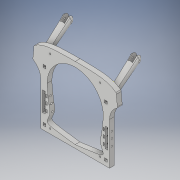
# Autodesk Inventor part: base
Saved by Autodesk Inventor 2019 (Build 230136000, 136)
## iProperties
Created: 2019-04-08
Part Number: base
Material: Ogólny
Document SubType Name: Modeling
Designer: terg
Density: 1 g/cm^3
Appearance: Domyślna
Author: terg
## iProperties of the stored document base_Drukowanie 3D.ipt
Created: 2019-04-08
Part Number: base_Drukowanie 3D
Material: Ogólny
Document SubType Name: Modeling
Designer: terg
Density: 1 g/cm^3
Appearance: Domyślna
Author: terg
Autodesk Inventor part; units mm, degrees
sketch "Szkic2" plane through (0, 0, 0) normal (0, 0, 1) x (1, 0, 0)
  line L0 (37, 65) -> (42, 65) construction
  line L1 (42, 28) -> (37, 28) construction
  line L2 (37, 65) -> (42, 65)
  line L3 (42, 65) -> (42, 28)
  line L4 (42, 28) -> (37, 28)
  line L5 (37, 28) -> (37, 65)
  line L6 (45, 80) -> (45, 0)
  line L7 (45, 0) -> (-20, 0)
  arc A0 (75, 110) -> (45, 80) centre (75, 80) ccw
  line L8 (75, 110) -> (77.9284, 114.3525) construction
  line L9 (77.9284, 114.3525) -> (81.9048, 129.5351) construction
  line L10 (81.9048, 129.5351) -> (73.952, 146.8867) construction
  line L11 (73.952, 146.8867) -> (59.3093, 153.7043) construction
  line L12 (59.3093, 153.7043) -> (47.9247, 160) construction
  line L13 (47.9247, 160) -> (-20, 160) construction
  spline S0 degree 4 poles (75, 110) (77.9284, 114.3525) (81.9048, 129.5351) (73.952, 146.8867) (59.3093, 153.7043) (47.9247, 160) (-20, 160) knots 1 1 1 1 1 2 3 4 4 4 4 4
  line L14 (0, 80) -> (0, 40) construction
  line L15 (-20, 0) -> (-20, 160) construction
  line L16 (-77, 65) -> (-82, 65) construction
  line L17 (-82, 28) -> (-77, 28) construction
  line L18 (-77, 65) -> (-82, 65)
  line L19 (-82, 65) -> (-82, 28)
  line L20 (-82, 28) -> (-77, 28)
  line L21 (-77, 28) -> (-77, 65)
  line L22 (-85, 80) -> (-85, 0)
  line L23 (-85, 0) -> (-20, 0)
  arc A1 (-85, 80) -> (-115, 110) centre (-115, 80) ccw
  line L24 (-115, 110) -> (-117.9284, 114.3525) construction
  line L25 (-117.9284, 114.3525) -> (-121.9048, 129.5351) construction
  line L26 (-121.9048, 129.5351) -> (-113.952, 146.8867) construction
  line L27 (-113.952, 146.8867) -> (-99.3093, 153.7043) construction
  line L28 (-99.3093, 153.7043) -> (-87.9247, 160) construction
  line L29 (-87.9247, 160) -> (-20, 160) construction
  spline S1 degree 4 poles (-115, 110) (-117.9284, 114.3525) (-121.9048, 129.5351) (-113.952, 146.8867) (-99.3093, 153.7043) (-87.9247, 160) (-20, 160) knots 1 1 1 1 1 2 3 4 4 4 4 4
  line L30 (-40, 80) -> (-40, 40) construction
  dimension "d23" = 30
  dimension "d24" = 65
  constraints: 38 end point, 21 symmetric about line, 8 coincident, 4 point on circle, 3 horizontal, 3 parallel, 2 centre point, 2 vertical, 1 perpendicular, 7 other
  measures "d23" radius of A0
  measures "d24" distance of L6.end L7.end
extrude "Wyciągnięcie proste1" add sketch "Szkic2" along normal blind 9
sketch "Szkic3" plane through (0, 0, 9) normal (0, 0, 1) x (1, 0, 0)
  line L0 (-85, 0) -> (45, 0) projected
  line L1 (-20, 0) -> (-67.244, 0)
  line L2 (-67.244, 0) -> (27.244, 0)
  circle A0 centre (-67.244, 8.994) radius 1.5
  circle A1 centre (27.244, 10) radius 1.5
  circle A2 centre (-67.244, 131.168) radius 1.5
  circle A3 centre (27.244, 131.168) radius 1.5
  point P0 (0, 0)
  dimension "d29" = 3
  dimension "d30" = 3
  dimension "d32" = 3
  dimension "d33" = 3
  constraints: 6 coincident, 4 centre point, 4 end point, 2 point on line, 1 midpoint
  measures "d29" diameter of A0
  measures "d30" diameter of A1
  measures "d32" diameter of A2
  measures "d33" diameter of A3
sketch "Szkic4" plane through (0, 0, 9) normal (0, 0, 1) x (1, 0, 0)
  line L0 (-85, 0) -> (45, 0) construction
  line L1 (-20, 0) -> (-20, 160) construction
  arc A0 (33.1064, 80) -> (-73.1064, 80) centre (-20, 80) ccw
  line L2 (-73.1064, 80) -> (-75.9423, 68.2413) construction
  line L3 (-75.9423, 68.2413) -> (-69.081, 45.3704) construction
  line L4 (-69.081, 45.3704) -> (-64.3162, 33.5537) construction
  line L5 (-64.3162, 33.5537) -> (-75.1799, 18.6876) construction
  line L6 (-75.1799, 18.6876) -> (-73.1064, 12.7793) construction
  line L7 (-73.1064, 12.7793) -> (-51.356, 10.6828) construction
  line L8 (-51.356, 10.6828) -> (-23.7203, 6.2992) construction
  line L9 (-23.7203, 6.2992) -> (-20, 6.2992) construction
  spline S0 degree 4 poles (-73.1064, 80) (-75.9423, 68.2413) (-69.081, 45.3704) (-64.3162, 33.5537) (-75.1799, 18.6876) (-73.1064, 12.7793) (-51.356, 10.6828) (-23.7203, 6.2992) (-20, 6.2992) knots 1 1 1 1 1 2 3 4 5 6 6 6 6 6
  line L10 (33.1064, 80) -> (35.9423, 68.2413) construction
  line L11 (35.9423, 68.2413) -> (29.081, 45.3704) construction
  line L12 (29.081, 45.3704) -> (24.3162, 33.5537) construction
  line L13 (24.3162, 33.5537) -> (35.1799, 18.6876) construction
  line L14 (35.1799, 18.6876) -> (33.1064, 12.7793) construction
  line L15 (33.1064, 12.7793) -> (11.356, 10.6828) construction
  line L16 (11.356, 10.6828) -> (-16.2797, 6.2992) construction
  line L17 (-16.2797, 6.2992) -> (-20, 6.2992) construction
  spline S1 degree 4 poles (33.1064, 80) (35.9423, 68.2413) (29.081, 45.3704) (24.3162, 33.5537) (35.1799, 18.6876) (33.1064, 12.7793) (11.356, 10.6828) (-16.2797, 6.2992) (-20, 6.2992) knots 1 1 1 1 1 2 3 4 5 6 6 6 6 6
  point P0 (0, 0)
  dimension "d34" = 160
  constraints: 7 symmetric about line, 2 end point, 2 midpoint, 2 point on circle, 1 centre point, 1 coincident, 1 perpendicular, 1 point on line, 1 vertical, 6 other
  measures "d34" distance of L1.start L1.end
extrude "Wyciągnięcie proste2" cut sketch "Szkic4" against normal blind 9
extrude "Wyciągnięcie proste3" cut sketch "Szkic3" against normal blind 9
sketch "Szkic5" plane through (0, 0, 9) normal (0, 0, 1) x (1, 0, 0)
  line L0 (-20, 160) -> (-20, 77.8902) construction
  line L1 (-20, 155) -> (-42.2049, 155) construction
  line L2 (-42.2049, 155) -> (-65.7509, 155) construction
  line L3 (-65.7509, 155) -> (-78.0422, 153.5632) construction
  line L4 (-78.0422, 153.5632) -> (-90.9908, 151.4994) construction
  line L5 (-90.9908, 151.4994) -> (-102.4767, 146.7512) construction
  line L6 (-102.4767, 146.7512) -> (-110.6216, 138.1137) construction
  line L7 (-110.6216, 138.1137) -> (-114.9161, 129.1287) construction
  line L8 (-114.9161, 129.1287) -> (-113.1391, 120.6877) construction
  line L9 (-113.1391, 120.6877) -> (-110.6216, 115.3565) construction
  spline S0 degree 4 poles (-20, 155) (-42.2049, 155) (-65.7509, 155) (-78.0422, 153.5632) (-90.9908, 151.4994) (-102.4767, 146.7512) (-110.6216, 138.1137) (-114.9161, 129.1287) (-113.1391, 120.6877) (-110.6216, 115.3565) knots 1 1 1 1 1 2 3 4 5 6 7 7 7 7 7
  line L10 (-110.6216, 115.3565) -> (-100.7117, 110.6199) construction
  line L11 (-100.7117, 110.6199) -> (-100.7117, 112.6806) construction
  line L12 (-100.7117, 112.6806) -> (-104.521, 114.5013) construction
  line L13 (-104.521, 114.5013) -> (-105.8067, 117.6302) construction
  line L14 (-105.8067, 117.6302) -> (-102.4767, 127.3399) construction
  line L15 (-102.4767, 127.3399) -> (-87.3718, 136.9774) construction
  line L16 (-87.3718, 136.9774) -> (-70.3325, 140.9019) construction
  line L17 (-70.3325, 140.9019) -> (-54.5401, 141.8394) construction
  line L18 (-54.5401, 141.8394) -> (-35.9852, 142.4325) construction
  line L19 (-35.9852, 142.4325) -> (-20, 142.4325) construction
  spline S1 degree 4 poles (-110.6216, 115.3565) (-100.7117, 110.6199) (-100.7117, 112.6806) (-104.521, 114.5013) (-105.8067, 117.6302) (-102.4767, 127.3399) (-87.3718, 136.9774) (-70.3325, 140.9019) (-54.5401, 141.8394) (-35.9852, 142.4325) (-20, 142.4325) knots 1 1 1 1 1 2 3 4 5 6 7 8 8 8 8 8
  line L20 (-20, 155) -> (2.2049, 155) construction
  line L21 (2.2049, 155) -> (25.7509, 155) construction
  line L22 (25.7509, 155) -> (38.0422, 153.5632) construction
  line L23 (38.0422, 153.5632) -> (50.9908, 151.4994) construction
  line L24 (50.9908, 151.4994) -> (62.4767, 146.7512) construction
  line L25 (62.4767, 146.7512) -> (70.6216, 138.1137) construction
  line L26 (70.6216, 138.1137) -> (74.9161, 129.1287) construction
  line L27 (74.9161, 129.1287) -> (73.1391, 120.6877) construction
  line L28 (73.1391, 120.6877) -> (70.6216, 115.3565) construction
  spline S2 degree 4 poles (-20, 155) (2.2049, 155) (25.7509, 155) (38.0422, 153.5632) (50.9908, 151.4994) (62.4767, 146.7512) (70.6216, 138.1137) (74.9161, 129.1287) (73.1391, 120.6877) (70.6216, 115.3565) knots 1 1 1 1 1 2 3 4 5 6 7 7 7 7 7
  line L29 (70.6216, 115.3565) -> (60.7117, 110.6199) construction
  line L30 (60.7117, 110.6199) -> (60.7117, 112.6806) construction
  line L31 (60.7117, 112.6806) -> (64.521, 114.5013) construction
  line L32 (64.521, 114.5013) -> (65.8067, 117.6302) construction
  line L33 (65.8067, 117.6302) -> (62.4767, 127.3399) construction
  line L34 (62.4767, 127.3399) -> (47.3718, 136.9774) construction
  line L35 (47.3718, 136.9774) -> (30.3325, 140.9019) construction
  line L36 (30.3325, 140.9019) -> (14.5401, 141.8394) construction
  line L37 (14.5401, 141.8394) -> (-4.0148, 142.4325) construction
  line L38 (-4.0148, 142.4325) -> (-20, 142.4325) construction
  spline S3 degree 4 poles (70.6216, 115.3565) (60.7117, 110.6199) (60.7117, 112.6806) (64.521, 114.5013) (65.8067, 117.6302) (62.4767, 127.3399) (47.3718, 136.9774) (30.3325, 140.9019) (14.5401, 141.8394) (-4.0148, 142.4325) (-20, 142.4325) knots 1 1 1 1 1 2 3 4 5 6 7 8 8 8 8 8
  point P0 (0, 0)
  constraints: 18 symmetric about line, 2 end point, 2 perpendicular, 2 point on line, 2 vertical, 12 other
extrude "Wyciągnięcie proste4" cut sketch "Szkic5" against normal blind 9
sketch "Szkic6" plane through (45, 0, 0) normal (1, 0, 0) x (0, 0, -1)
  line L0 (-9, 28) -> (-9, 65) projected
  line L1 (0, 65) -> (0, 28) projected
  line L2 (0, 28) -> (-9, 28) construction
  line L3 (-9, 28) -> (0, 28) construction
  line L4 (0, 65) -> (-9, 65) construction
  line L5 (0, 65) -> (-9, 65) construction
  line L6 (-4.5, 28) -> (-4.5, 34) construction
  circle A0 centre (-4.5, 34) radius 1.5
  line L7 (-4.5, 34) -> (-4.5, 46.5) construction
  circle A1 centre (-4.5, 46.5) radius 1.5
  line L8 (-4.5, 46.5) -> (-4.5, 58.5) construction
  circle A2 centre (-4.5, 58.5) radius 1.5
  point P0 (0, 0)
  dimension "d41" = 6
  dimension "d42" = 3
  dimension "d43" = 12.5
  dimension "d44" = 3
  dimension "d45" = 12
  dimension "d46" = 3
  constraints: 10 end point, 3 centre point, 3 coincident, 3 vertical, 1 collinear, 1 horizontal, 1 midpoint
  measures "d41" distance of L6.start L6.end
  measures "d42" diameter of A0
  measures "d43" distance of L7.start L7.end
  measures "d44" diameter of A1
  measures "d45" distance of L8.start L8.end
  measures "d46" diameter of A2
extrude "Wyciągnięcie proste5" cut sketch "Szkic6" against normal blind 11
ref_plane "Płaszczyzna konstrukcyjna1" through (-20, 0, 0) normal (1, 0, 0) x (0, 1, 0)
mirror "Odbij1" about plane through (-20, 0, 0) normal (1, 0, 0) of "Wyciągnięcie proste5"
sketch "Szkic7" plane through (0, 0, 9) normal (0, 0, 1) x (1, 0, 0)
  line L0 (37, 35.5) -> (37, 32.5) projected
  line L1 (37, 48) -> (37, 45) projected
  line L2 (37, 60) -> (37, 57) projected
  line L3 (37, 58.5) -> (27.7533, 58.5) construction
  line L4 (37, 46.5) -> (27.7533, 46.5) construction
  line L5 (37, 34) -> (27.7533, 34) construction
  line L6 (33.1, 43.75) -> (35.4, 43.75)
  line L7 (35.4, 43.75) -> (35.4, 49.25)
  line L8 (35.4, 49.25) -> (33.1, 49.25)
  line L9 (33.1, 49.25) -> (33.1, 43.75)
  line L10 (33.1, 43.75) -> (35.4, 49.25) construction
  line L11 (35.4, 43.75) -> (33.1, 49.25) construction
  line L12 (33.1, 31.25) -> (35.4, 31.25)
  line L13 (35.4, 31.25) -> (35.4, 36.75)
  line L14 (35.4, 36.75) -> (33.1, 36.75)
  line L15 (33.1, 36.75) -> (33.1, 31.25)
  line L16 (33.1, 31.25) -> (35.4, 36.75) construction
  line L17 (35.4, 31.25) -> (33.1, 36.75) construction
  line L18 (33, 55.75) -> (35.5, 55.75)
  line L19 (35.5, 55.75) -> (35.5, 61.25)
  line L20 (35.5, 61.25) -> (33, 61.25)
  line L21 (33, 61.25) -> (33, 55.75)
  line L22 (33, 55.75) -> (35.5, 61.25) construction
  line L23 (35.5, 55.75) -> (33, 61.25) construction
  spline S0 degree 4 poles (33.1064, 80) (35.9423, 68.2413) (29.081, 45.3704) (24.3162, 33.5537) (35.1799, 18.6876) (33.1064, 12.7793) (11.356, 10.6828) (-16.2797, 6.2992) (-20, 6.2992) knots 0 0 0 0 0 0.2 0.4 0.6 0.8 1 1 1 1 1 projected
  line L24 (29.4637, 46.5) -> (30.5401, 52.1183) construction
  line L25 (30.5401, 52.1183) -> (31.3941, 62.4324) construction
  line L26 (31.3941, 62.4324) -> (33.1064, 73.5348) construction
  line L27 (33.1064, 73.5348) -> (33.1064, 80) construction
  spline S1 degree 4 poles (29.4637, 46.5) (30.5401, 52.1183) (31.3941, 62.4324) (33.1064, 73.5348) (33.1064, 80) knots 1 1 1 1 1 2 2 2 2 2
  point P0 (0, 0)
  point P1 (34.25, 58.5)
  point P2 (34.25, 46.5)
  point P3 (34.25, 34)
  dimension "d50" = 2.3
  dimension "d51" = 5.5
  dimension "d52" = 2.3
  dimension "d53" = 5.5
  dimension "d54" = 2.5
  dimension "d55" = 5.5
  constraints: 42 end point, 9 midpoint, 6 horizontal, 6 parallel, 4 point on line, 3 perpendicular, 1 coincident, 1 vertical, 6 other
  measures "d50" distance of L8.end L7.end
  measures "d51" distance of L7.end L6.end
  measures "d52" distance of L14.end L13.end
  measures "d53" distance of L13.end L12.end
  measures "d54" distance of L20.end L19.end
  measures "d55" distance of L19.end L18.end
extrude "Wyciągnięcie proste6" add sketch "Szkic7" against normal blind 9 contours S0 S1 L20 L21 | L21 L20 S0
extrude "Wyciągnięcie proste7" cut sketch "Szkic7" against normal blind 9 contours L9 L8 L7 L6 | L15 L14 L13 L12 | L21 S0 L20 L19 L18 | L21 L20 S0
sketch "Szkic8" plane through (45, 0, 0) normal (1, 0, 0) x (0, 0, -1)
  circle A0 centre (-4.5, 34) radius 1.5 projected
  circle A1 centre (-4.5, 46.5) radius 1.5 projected
  circle A2 centre (-4.5, 58.5) radius 1.5 projected
  point P0 (0, 0)
extrude "Wyciągnięcie proste8" cut sketch "Szkic8" against normal blind 20
mirror "Odbij2" about plane through (-20, 0, 0) normal (1, 0, 0) of "Wyciągnięcie proste6", "Wyciągnięcie proste7", "Wyciągnięcie proste8"
sketch "Szkic9" plane through (0, 0, 0) normal (0, 0, -1) x (-1, 0, 0)
  line L0 (75.4, 36.75) -> (75.4, 31.25) construction
  line L1 (75.4, 31.25) -> (73.1, 31.25) construction
  line L2 (73.1, 31.25) -> (73.1, 36.75) construction
  line L3 (73.1, 36.75) -> (75.4, 36.75) construction
  line L4 (75.4, 49.25) -> (75.4, 43.75) construction
  line L5 (75.4, 43.75) -> (73.1, 43.75) construction
  line L6 (73.1, 43.75) -> (73.1, 49.25) construction
  line L7 (73.1, 49.25) -> (75.4, 49.25) construction
  line L8 (75.5, 61.25) -> (75.5, 55.75) construction
  line L9 (75.5, 55.75) -> (73, 55.75) construction
  line L10 (73, 55.75) -> (73, 61.25) construction
  line L11 (73, 61.25) -> (75.5, 61.25) construction
  line L12 (-35.5, 55.75) -> (-35.5, 61.25) construction
  line L13 (-35.5, 61.25) -> (-33, 61.25) construction
  line L14 (-33, 61.25) -> (-33, 55.75) construction
  line L15 (-33, 55.75) -> (-35.5, 55.75) construction
  line L16 (-35.4, 43.75) -> (-35.4, 49.25) construction
  line L17 (-35.4, 49.25) -> (-33.1, 49.25) construction
  line L18 (-33.1, 49.25) -> (-33.1, 43.75) construction
  line L19 (-33.1, 43.75) -> (-35.4, 43.75) construction
  line L20 (-35.4, 31.25) -> (-35.4, 36.75) construction
  line L21 (-35.4, 36.75) -> (-33.1, 36.75) construction
  line L22 (-33.1, 36.75) -> (-33.1, 31.25) construction
  line L23 (-33.1, 31.25) -> (-35.4, 31.25) construction
  circle A0 centre (67.244, 131.168) radius 1.5 construction
  circle A1 centre (67.244, 8.994) radius 1.5 construction
  circle A2 centre (-27.244, 10) radius 1.5 construction
  circle A3 centre (-27.244, 131.168) radius 1.5 construction
  arc A4 (73.1064, 80) -> (-33.1064, 80) centre (20, 80) ccw construction
  line L24 (77, 28) -> (77, 65) construction
  line L25 (77, 65) -> (82, 65) construction
  line L26 (82, 65) -> (82, 28) construction
  line L27 (82, 28) -> (77, 28) construction
  line L28 (-42, 28) -> (-42, 65) construction
  line L29 (-42, 65) -> (-37, 65) construction
  line L30 (-37, 65) -> (-37, 28) construction
  line L31 (-37, 28) -> (-42, 28) construction
  line L32 (85, 0) -> (-45, 0) construction
  line L33 (85, 80) -> (85, 0) construction
  arc A5 (115, 110) -> (85, 80) centre (115, 80) ccw construction
  arc A6 (-45, 80) -> (-75, 110) centre (-75, 80) ccw construction
  line L34 (-45, 0) -> (-45, 80) construction
  line L35 (-49.3106, 116.6116) -> (-39.3106, 116.6116)
  line L36 (-39.3106, 116.6116) -> (-39.3106, 126.6116)
  line L37 (-39.3106, 126.6116) -> (-49.3106, 126.6116)
  line L38 (-49.3106, 126.6116) -> (-49.3106, 116.6116)
  line L39 (-49.3106, 116.6116) -> (-39.3106, 126.6116) construction
  line L40 (-39.3106, 116.6116) -> (-49.3106, 126.6116) construction
  point P0 (0, 0)
  point P1 (-44.3106, 121.6116)
  dimension "d62" = 10
  dimension "d63" = 10
  constraints: 12 end point, 2 midpoint, 2 parallel, 1 horizontal, 1 perpendicular, 10 other
  measures "d62" distance of L37.end L36.end
  measures "d63" distance of L36.end L35.end
ref_plane "Płaszczyzna konstrukcyjna3" through (0, 0, -39.5) normal (0, 0, -1) x (-1, 0, 0)
ref_plane "Płaszczyzna konstrukcyjna5" through (52.8106, 146.0683, -39.5) normal (0, 0, -1) x (-1, 0, 0)
sketch "Szkic12" plane through (52.8106, 146.0683, -39.5) normal (0, 0, -1) x (-1, 0, 0)
  line L0 (0, 0) -> (17, 0) projected
  line L1 (17, 0) -> (17, 17) projected
  line L2 (17, 17) -> (0, 17) projected
  line L3 (0, 17) -> (0, 0) projected
  line L4 (0, 0) -> (17, 0) projected
  line L5 (8.5, 0) -> (8.5, 17)
  arc A0 (8.5, 0) -> (8.5, 17) centre (8.5, 8.5) ccw
  point P0 (52.8106, -146.0683)
  constraints: 2 end point, 2 midpoint, 2 point on circle, 1 centre point, 1 tangent
revolve "Obrót1" add sketch "Szkic12" angle 180 about axis through (44.3106, 146.0683, -39.5) along (0, -1, 0) contours L5 A0
loft "Wyciągnięcie złożone2" add profiles "Szkic9" section 2 edges at (35.8106, 154.5683, -39.5) (52.8106, 154.5683, -39.5)
mirror "Odbij3" about plane through (-20, 0, 0) normal (1, 0, 0) of "Wyciągnięcie złożone2", "Obrót1"
sketch "Szkic13" plane through (0, 0, 9) normal (0, 0, 1) x (1, 0, 0)
  line L0 (-89.3106, 116.6116) -> (-79.3106, 116.6116) projected
  line L1 (-79.3106, 116.6116) -> (-79.3106, 126.6116) projected
  line L2 (-79.3106, 126.6116) -> (-89.3106, 126.6116) projected
  line L3 (-89.3106, 126.6116) -> (-89.3106, 116.6116) projected
  line L4 (39.3106, 116.6116) -> (49.3106, 116.6116) projected
  line L5 (49.3106, 116.6116) -> (49.3106, 126.6116) projected
  line L6 (49.3106, 126.6116) -> (39.3106, 126.6116) projected
  line L7 (39.3106, 126.6116) -> (39.3106, 116.6116) projected
  line L8 (-75.4, 36.75) -> (-75.4, 31.25) projected
  line L9 (-75.4, 31.25) -> (-73.1, 31.25) projected
  line L10 (-73.1, 31.25) -> (-73.1, 36.75) projected
  line L11 (-73.1, 36.75) -> (-75.4, 36.75) projected
  line L12 (-75.4, 49.25) -> (-75.4, 43.75) projected
  line L13 (-75.4, 43.75) -> (-73.1, 43.75) projected
  line L14 (-73.1, 43.75) -> (-73.1, 49.25) projected
  line L15 (-73.1, 49.25) -> (-75.4, 49.25) projected
  line L16 (-75.5, 61.25) -> (-75.5, 55.75) projected
  line L17 (-75.5, 55.75) -> (-73, 55.75) projected
  line L18 (-73, 55.75) -> (-73, 61.25) projected
  line L19 (-73, 61.25) -> (-75.5, 61.25) projected
  line L20 (35.5, 55.75) -> (35.5, 61.25) projected
  line L21 (35.5, 61.25) -> (33, 61.25) projected
  line L22 (33, 61.25) -> (33, 55.75) projected
  line L23 (33, 55.75) -> (35.5, 55.75) projected
  line L24 (35.4, 43.75) -> (35.4, 49.25) projected
  line L25 (35.4, 49.25) -> (33.1, 49.25) projected
  line L26 (33.1, 49.25) -> (33.1, 43.75) projected
  line L27 (33.1, 43.75) -> (35.4, 43.75) projected
  line L28 (35.4, 31.25) -> (35.4, 36.75) projected
  line L29 (35.4, 36.75) -> (33.1, 36.75) projected
  line L30 (33.1, 36.75) -> (33.1, 31.25) projected
  line L31 (33.1, 31.25) -> (35.4, 31.25) projected
  circle A0 centre (-67.244, 131.168) radius 1.5 projected
  circle A1 centre (-67.244, 8.994) radius 1.5 projected
  circle A2 centre (27.244, 10) radius 1.5 projected
  circle A3 centre (27.244, 131.168) radius 1.5 projected
  arc A4 (33.1064, 80) -> (-73.1064, 80) centre (-20, 80) ccw projected
  line L32 (-77, 28) -> (-77, 65) projected
  line L33 (-77, 65) -> (-82, 65) projected
  line L34 (-82, 65) -> (-82, 28) projected
  line L35 (-82, 28) -> (-77, 28) projected
  line L36 (42, 28) -> (42, 65) projected
  line L37 (42, 65) -> (37, 65) projected
  line L38 (37, 65) -> (37, 28) projected
  line L39 (37, 28) -> (42, 28) projected
  line L40 (-85, 0) -> (45, 0) projected
  line L41 (-85, 80) -> (-85, 0) projected
  arc A5 (-85, 80) -> (-115, 110) centre (-115, 80) ccw projected
  arc A6 (75, 110) -> (45, 80) centre (75, 80) ccw projected
  line L42 (45, 0) -> (45, 80) projected
  line L43 (-75.4, 31.25) -> (-75.4, 36.75) projected
  line L44 (-75.4, 36.75) -> (-73.1, 36.75) projected
  line L45 (-73.1, 36.75) -> (-73.1, 31.25) projected
  line L46 (-73.1, 31.25) -> (-75.4, 31.25) projected
  line L47 (-75.4, 43.75) -> (-75.4, 49.25) projected
  line L48 (-75.4, 49.25) -> (-73.1, 49.25) projected
  line L49 (-73.1, 49.25) -> (-73.1, 43.75) projected
  line L50 (-73.1, 43.75) -> (-75.4, 43.75) projected
  line L51 (-75.5, 55.75) -> (-75.5, 61.25) projected
  line L52 (-75.5, 61.25) -> (-73, 61.25) projected
  line L53 (-73, 61.25) -> (-73, 55.75) projected
  line L54 (-73, 55.75) -> (-75.5, 55.75) projected
  line L55 (35.5, 61.25) -> (35.5, 55.75) projected
  line L56 (35.5, 55.75) -> (33, 55.75) projected
  line L57 (33, 55.75) -> (33, 61.25) projected
  line L58 (33, 61.25) -> (35.5, 61.25) projected
  line L59 (35.4, 49.25) -> (35.4, 43.75) projected
  line L60 (35.4, 43.75) -> (33.1, 43.75) projected
  line L61 (33.1, 43.75) -> (33.1, 49.25) projected
  line L62 (33.1, 49.25) -> (35.4, 49.25) projected
  line L63 (35.4, 36.75) -> (35.4, 31.25) projected
  line L64 (35.4, 31.25) -> (33.1, 31.25) projected
  line L65 (33.1, 31.25) -> (33.1, 36.75) projected
  line L66 (33.1, 36.75) -> (35.4, 36.75) projected
  circle A7 centre (-67.244, 131.168) radius 1.5 projected
  circle A8 centre (-67.244, 8.994) radius 1.5 projected
  circle A9 centre (27.244, 10) radius 1.5 projected
  circle A10 centre (27.244, 131.168) radius 1.5 projected
  arc A11 (33.1064, 80) -> (-73.1064, 80) centre (-20, 80) ccw projected
  line L67 (-77, 65) -> (-77, 28) projected
  line L68 (-77, 28) -> (-82, 28) projected
  line L69 (-82, 28) -> (-82, 65) projected
  line L70 (-82, 65) -> (-77, 65) projected
  line L71 (42, 65) -> (42, 28) projected
  line L72 (42, 28) -> (37, 28) projected
  line L73 (37, 28) -> (37, 65) projected
  line L74 (37, 65) -> (42, 65) projected
  line L75 (-85, 0) -> (45, 0) projected
  line L76 (45, 0) -> (45, 80) projected
  arc A12 (75, 110) -> (45, 80) centre (75, 80) ccw projected
  arc A13 (-85, 80) -> (-115, 110) centre (-115, 80) ccw projected
  line L77 (-85, 80) -> (-85, 0) projected
  line L78 (45, 0) -> (38, 0) construction
  line L79 (38, 0) -> (38, 10) construction
  line L80 (38, 10) -> (45, 10) construction
  line L81 (45, 10) -> (45, 0) construction
  line L82 (35.5, 12.5) -> (40.5, 12.5)
  line L83 (40.5, 12.5) -> (40.5, 7.5)
  line L84 (40.5, 7.5) -> (35.5, 7.5)
  line L85 (35.5, 7.5) -> (35.5, 12.5)
  line L86 (35.5, 12.5) -> (40.5, 7.5) construction
  line L87 (40.5, 12.5) -> (35.5, 7.5) construction
  line L88 (38, 10) -> (38, 105) construction
  line L89 (35.5, 107.5) -> (40.5, 107.5)
  line L90 (40.5, 107.5) -> (40.5, 102.5)
  line L91 (40.5, 102.5) -> (35.5, 102.5)
  line L92 (35.5, 102.5) -> (35.5, 107.5)
  line L93 (35.5, 107.5) -> (40.5, 102.5) construction
  line L94 (40.5, 107.5) -> (35.5, 102.5) construction
  point P0 (0, 0)
  dimension "d79" = 7
  dimension "d80" = 10
  dimension "d81" = 5
  dimension "d82" = 5
  dimension "d83" = 95
  dimension "d84" = 5
  dimension "d85" = 5
  constraints: 34 end point, 6 parallel, 4 midpoint, 3 horizontal, 3 perpendicular, 1 vertical, 20 other
  measures "d79" distance of L79.end L80.end
  measures "d80" distance of L78.end L79.end
  measures "d81" distance of L83.end L84.end
  measures "d82" distance of L82.end L83.end
  measures "d83" distance of L79.end L88.end
  measures "d84" distance of L90.end L91.end
  measures "d85" distance of L89.end L90.end
extrude "Wyciągnięcie proste9" cut sketch "Szkic13" against normal blind 20 contours L82 L83 L84 L85 | L89 L90 L91 L92
mirror "Odbij4" about plane through (-20, 0, 0) normal (1, 0, 0) of "Wyciągnięcie proste9"
sketch "Szkic14" plane through (0, 0, 0) normal (0, 0, -1) x (-1, 0, 0)
  point P0 (0, 0)
sketch "Szkic15" plane through (0, 0, 0) normal (0, 0, -1) x (-1, 0, 0)
  line L0 (75.5, 7.5) -> (75.5, 12.5) projected
  line L1 (75.5, 12.5) -> (80.5, 12.5) projected
  line L2 (80.5, 12.5) -> (80.5, 7.5) projected
  line L3 (80.5, 7.5) -> (75.5, 7.5) projected
  line L4 (75.5, 102.5) -> (75.5, 107.5) projected
  line L5 (75.5, 107.5) -> (80.5, 107.5) projected
  line L6 (80.5, 107.5) -> (80.5, 102.5) projected
  line L7 (80.5, 102.5) -> (75.5, 102.5) projected
  line L8 (-35.5, 12.5) -> (-35.5, 7.5) projected
  line L9 (-35.5, 7.5) -> (-40.5, 7.5) projected
  line L10 (-40.5, 7.5) -> (-40.5, 12.5) projected
  line L11 (-40.5, 12.5) -> (-35.5, 12.5) projected
  line L12 (-35.5, 107.5) -> (-35.5, 102.5) projected
  line L13 (-35.5, 102.5) -> (-40.5, 102.5) projected
  line L14 (-40.5, 102.5) -> (-40.5, 107.5) projected
  line L15 (-40.5, 107.5) -> (-35.5, 107.5) projected
  line L16 (75.4, 36.75) -> (75.4, 31.25) projected
  line L17 (75.4, 31.25) -> (73.1, 31.25) projected
  line L18 (73.1, 31.25) -> (73.1, 36.75) projected
  line L19 (73.1, 36.75) -> (75.4, 36.75) projected
  line L20 (75.4, 49.25) -> (75.4, 43.75) projected
  line L21 (75.4, 43.75) -> (73.1, 43.75) projected
  line L22 (73.1, 43.75) -> (73.1, 49.25) projected
  line L23 (73.1, 49.25) -> (75.4, 49.25) projected
  line L24 (75.5, 61.25) -> (75.5, 55.75) projected
  line L25 (75.5, 55.75) -> (73, 55.75) projected
  line L26 (73, 55.75) -> (73, 61.25) projected
  line L27 (73, 61.25) -> (75.5, 61.25) projected
  line L28 (-35.5, 55.75) -> (-35.5, 61.25) projected
  line L29 (-35.5, 61.25) -> (-33, 61.25) projected
  line L30 (-33, 61.25) -> (-33, 55.75) projected
  line L31 (-33, 55.75) -> (-35.5, 55.75) projected
  line L32 (-35.4, 43.75) -> (-35.4, 49.25) projected
  line L33 (-35.4, 49.25) -> (-33.1, 49.25) projected
  line L34 (-33.1, 49.25) -> (-33.1, 43.75) projected
  line L35 (-33.1, 43.75) -> (-35.4, 43.75) projected
  line L36 (-35.4, 31.25) -> (-35.4, 36.75) projected
  line L37 (-35.4, 36.75) -> (-33.1, 36.75) projected
  line L38 (-33.1, 36.75) -> (-33.1, 31.25) projected
  line L39 (-33.1, 31.25) -> (-35.4, 31.25) projected
  circle A0 centre (67.244, 131.168) radius 1.5 projected
  circle A1 centre (67.244, 8.994) radius 1.5 projected
  circle A2 centre (-27.244, 10) radius 1.5 projected
  circle A3 centre (-27.244, 131.168) radius 1.5 projected
  arc A4 (73.1064, 80) -> (-33.1064, 80) centre (20, 80) ccw projected
  line L40 (77, 28) -> (77, 65) projected
  line L41 (77, 65) -> (82, 65) projected
  line L42 (82, 65) -> (82, 28) projected
  line L43 (82, 28) -> (77, 28) projected
  line L44 (-42, 28) -> (-42, 65) projected
  line L45 (-42, 65) -> (-37, 65) projected
  line L46 (-37, 65) -> (-37, 28) projected
  line L47 (-37, 28) -> (-42, 28) projected
  line L48 (85, 0) -> (-45, 0) projected
  line L49 (85, 80) -> (85, 0) projected
  arc A5 (115, 110) -> (85, 80) centre (115, 80) ccw projected
  spline S0 degree 4 poles (-75, 110) (-77.9284, 114.3525) (-81.9048, 129.5351) (-73.952, 146.8867) (-59.3093, 153.7043) (-47.9247, 160) (20, 160) knots 0 0 0 0 0 0.333333 0.666667 1 1 1 1 1 projected
  arc A6 (-45, 80) -> (-75, 110) centre (-75, 80) ccw projected
  line L50 (-45, 0) -> (-45, 80) projected
  line L51 (-60.3524, 106.1811) -> (-60.3524, 153.0565) construction
  arc A7 (-60.3524, 106.1811) -> (-60.3524, 153.0565) centre (-182.6787, 129.6188) ccw
  arc A8 (-60.3524, 153.0565) -> (-60.3524, 106.1811) centre (-75.3663, 129.6188) ccw
  point P0 (0, 0)
  constraints: 5 point on circle, 4 horizontal alignment, 4 vertical alignment, 2 centre point, 2 end point, 1 vertical, 13 other
extrude "Wyciągnięcie proste10" cut sketch "Szkic15" against normal blind 20 contours S0 A7 A6
mirror "Odbij5" about plane through (-20, 0, 0) normal (1, 0, 0) of "Wyciągnięcie proste10"
sketch "Szkic16" plane through (0, 0, 0) normal (0, 0, -1) x (-1, 0, 0)
  line L0 (116.1445, 195.8948) -> (-69.6162, 195.8948)
  line L1 (-69.6162, 195.8948) -> (-69.6162, 145.1366)
  line L2 (-69.6162, 145.1366) -> (116.1445, 145.1366)
  line L3 (116.1445, 145.1366) -> (116.1445, 195.8948)
  line L4 (116.1445, 195.8948) -> (-69.6162, 145.1366) construction
  line L5 (-69.6162, 195.8948) -> (116.1445, 145.1366) construction
  point P0 (0, 0)
  point P1 (23.2642, 170.5157)
  constraints: 12 end point, 2 midpoint, 2 parallel, 1 horizontal, 1 perpendicular
extrude "Wyciągnięcie proste11" cut sketch "Szkic16" against normal blind 20
fillet "Zaokrąglenie2" radius 3 4 edges at (60.3524, 106.1811, 4.5) (58.1282, 129.1339, 4.5) (-100.3524, 106.1811, 4.5) (-98.1282, 129.1339, 4.5)
sketch "Szkic17" plane through (-20, 0, 0) normal (1, 0, 0) x (0, 1, 0)
  point P0 (0, 0)
sketch "Szkic18" plane through (-20, 0, 0) normal (1, 0, 0) x (0, 1, 0)
  arc A0 (146.0683, -39.5) -> (163.0683, -39.5) centre (154.5683, -39.5) ccw construction
  line L0 (80, 9) -> (105.1612, 9) construction
  line L1 (163.0683, 9) -> (0, 9) construction
  line L2 (0, 9) -> (0, -48) construction
  line L3 (0, -48) -> (163.0683, -48) construction
  line L4 (163.0683, -48) -> (163.0683, 9) construction
  point P0 (0, 0)
  constraints: 8 end point, 2 parallel, 1 horizontal, 1 perpendicular
sketch "Szkic19" plane through (-20, 0, 0) normal (1, 0, 0) x (0, 1, 0)
  point P0 (0, 0)
sketch "Szkic20" plane through (0, 0, 0) normal (0, 0, -1) x (-1, 0, 0)
  line L0 (-44.3106, 116.6116) -> (-44.3106, 138.9305) construction
  point P0 (0, 0)
  constraints: 2 end point, 1 vertical, 2 other
ref_plane "Płaszczyzna konstrukcyjna6" through (44.3106, 116.6116, 0) normal (1, 0, 0) x (0, 1, 0)
sketch "Szkic21" plane through (44.3106, 116.6116, 0) normal (1, 0, 0) x (0, 1, 0)
  arc A0 (29.4567, -39.5) -> (46.4567, -39.5) centre (37.9567, -39.5) ccw projected
  line L0 (46.4567, -39.5) -> (29.4567, -39.5) construction
  arc A1 (46.4567, -39.5) -> (29.4567, -39.5) centre (37.9567, -39.5) ccw
  point P0 (-116.6116, 0)
  constraints: 2 end point, 2 point on circle, 1 centre point, 1 horizontal, 1 other
extrude "Wyciągnięcie proste12" cut sketch "Szkic21" along normal mid plane 8
sketch "Szkic22" plane through (44.3106, 116.6116, 0) normal (1, 0, 0) x (0, 1, 0)
  arc A0 (30.4567, -39.5) -> (43.9671, -39.5) centre (37.9567, -39.5) ccw construction
  line L0 (43.9671, -39.5) -> (37.0649, -39.5) construction
  line L1 (37.0649, -39.5) -> (37.0649, -39.5) construction
  line L2 (37.0649, -39.5) -> (31.9462, -39.5) construction
  line L3 (31.9462, -39.5) -> (30.4567, -39.5) construction
  arc A1 (30.4567, -39.5) -> (43.9671, -39.5) centre (37.9567, -39.5) ccw construction
  line L4 (37.0649, -39.5) -> (43.9671, -39.5) construction
  line L5 (43.9671, -39.5) -> (30.4567, -39.5) construction
  circle A2 centre (37.9567, -39.5) radius 1.5
  point P0 (-116.6116, 0)
  dimension "d95" = 3
  constraints: 2 coincident, 2 end point, 1 centre point, 1 collinear, 2 other
  measures "d95" diameter of A2
extrude "Wyciągnięcie proste13" cut sketch "Szkic22" along normal blind 200 and the other way blind 300
mirror "Odbij6" about plane through (-20, 0, 0) normal (1, 0, 0) of "Wyciągnięcie proste12"
